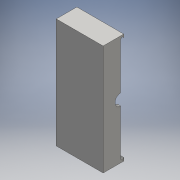
# Autodesk Inventor part: Pieza1
Saved by Autodesk Inventor 2016 (Build 200138000, 138)
## iProperties
Created: 2016-10-17
Part Number: Pieza1
Material: Genérico
Document SubType Name: Modeling
Designer: Roberto
Density: 1 g/cm^3
Appearance: Valor por defecto
Author: Roberto
Autodesk Inventor part; units mm, degrees
ref_plane "YZ Plane" through (0, 0, 0) normal (1, 0, 0) x (0, 1, 0)
ref_plane "XZ Plane" through (0, 0, 0) normal (0, 1, 0) x (-1, 0, 0)
ref_plane "XY Plane" through (0, 0, 0) normal (0, 0, 1) x (1, 0, 0)
sketch "Boceto1" plane through (0, 0, 0) normal (0, 1, 0) x (-1, 0, 0)
  line L0 (0, 0) -> (0, -17.6)
  line L1 (0, -17.6) -> (7.5, -17.6)
  line L2 (7.5, -17.6) -> (7.5, 0)
  line L3 (7.5, 0) -> (0, 0)
  dimension "d0" = 17.6
  dimension "d1" = 7.5
  constraints: 8 end point, 3 perpendicular, 1 vertical
  measures "d0" distance of L0.start L0.end
  measures "d1" distance of L0.end L1.end
extrude "Extrusión1" add sketch "Boceto1" along normal blind 3.3
sketch "Boceto2" plane through (0, 3.3, 0) normal (0, 1, 0) x (1, 0, 0)
  line L0 (0, 0) -> (0, 17.6) projected
  line L1 (0, 17.6) -> (-7.5, 17.6) projected
  line L2 (-7.5, 17.6) -> (-7.5, 0) projected
  line L3 (-7.5, 0) -> (0, 0) projected
  line L4 (-7, 0.5) -> (-7, 17.1)
  line L5 (-7, 17.1) -> (-0.5, 17.1)
  line L6 (-0.5, 17.1) -> (-0.5, 0.5)
  line L7 (-0.5, 0.5) -> (-7, 0.5)
  dimension "d4" = 0.5
  constraints: 8 end point, 3 other
  measures "d4" distance between parallel lines of L2 L4
extrude "Extrusión2" cut sketch "Boceto2" against normal blind 2.8 contours L4 L5 L6 L7
sketch "Boceto3" plane through (0, 3.3, 0) normal (0, 1, 0) x (1, 0, 0)
  line L0 (-0.5, 17.1) -> (-0.5, 0.5) projected
  line L1 (-0.5, 0.5) -> (0, 0.5)
  line L2 (0, 0.5) -> (0, 17.1)
  line L3 (0, 0) -> (0, 17.6) projected
  line L4 (-0.5, 17.1) -> (-0.5, 0.5) projected
  line L5 (-0.5, 17.1) -> (-0.5, 0.5)
  line L6 (-0.5, 0.5) -> (-0.5, 17.1)
  line L7 (-0.5, 17.1) -> (0, 17.1)
  constraints: 10 end point, 1 collinear, 1 horizontal, 1 perpendicular, 1 point on line, 1 vertical
extrude "Extrusión3" cut sketch "Boceto3" against normal blind 0.5
sketch "Boceto4" plane through (0, 0, 0) normal (1, 0, 0) x (0, 0, -1)
  line L0 (0.5, 2.8) -> (0.5, 3.3) projected
  line L1 (0, 3.3) -> (0.5, 3.3) projected
  line L2 (0, 0) -> (0, 3.3) projected
  line L3 (0, 0) -> (17.6, 0) projected
  line L4 (17.6, 0) -> (17.6, 3.3) projected
  line L5 (17.1, 3.3) -> (17.6, 3.3) projected
  line L6 (17.1, 3.3) -> (17.1, 2.8) projected
  line L7 (17.1, 2.8) -> (0.5, 2.8) projected
  line L8 (0.5, 3.3) -> (0.5, 0.5) projected
  line L9 (0.5, 2.8) -> (0.5, 3.3)
  line L10 (0.5, 3.3) -> (0.5, 3.05)
  line L11 (0.5, 2.8) -> (0.25, 3.05)
  line L12 (0.5, 3.3) -> (0.25, 3.05)
  line L13 (17.1, 3.3) -> (17.1, 2.8)
  line L14 (17.1, 3.3) -> (17.6, 3.3) projected
  line L15 (17.1, 3.3) -> (17.35, 3.05)
  line L16 (17.35, 3.05) -> (17.1, 2.8)
  constraints: 14 end point, 3 perpendicular, 1 collinear, 1 midpoint
extrude "Extrusión4" cut sketch "Boceto4" against normal blind 7 contours L11 L12 L0 | L6 L15 L16
sketch "Boceto5" plane through (0, 0, 0) normal (1, 0, 0) x (0, 0, -1)
  line L0 (0.5, 2.8) -> (17.1, 2.8) projected
  circle A0 centre (8.8, 2.8) radius 0.9
  line L1 (7.9, 2.8) -> (9.7, 2.8)
  point P0 (0, 0)
  dimension "d11" = 1.8
  constraints: 2 end point, 2 point on circle, 2 point on line, 1 centre point, 1 midpoint
  measures "d11" diameter of A0
extrude "Extrusión5" cut sketch "Boceto5" against normal blind 5 contours L0 A0 picked at (8.728, 2.3801)
